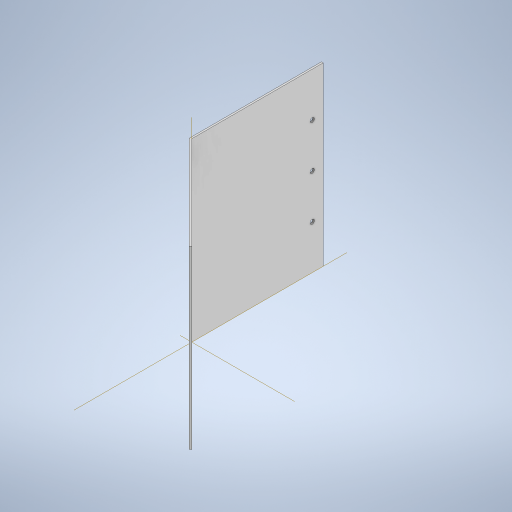
# Autodesk Inventor part: Thesis_part
Saved by Autodesk Inventor 2024 (Build 280153000, 153)
## iProperties
Created: 2024-02-06
Part Number: Thesis_part
Material: Generic
Document SubType Name: Modeling
Designer: Administrator
Density: 1 g/cm^3
Appearance: Default
Author: Administrator
Autodesk Inventor part; units mm, degrees
ref_plane "YZ Plane" through (0, 0, 0) normal (1, 0, 0) x (0, 1, 0)
ref_plane "XZ Plane" through (0, 0, 0) normal (0, 1, 0) x (-1, 0, 0)
ref_plane "XY Plane" through (0, 0, 0) normal (0, 0, 1) x (1, 0, 0)
sketch "Sketch2" plane through (0, 0, 0) normal (0, 1, 0) x (-1, 0, 0)
  line L0 (0, 0) -> (0, -149.1716)
  line L1 (-105.4802, 105.4802) -> (0, 0)
  line L2 (2, 0.8284) -> (2, -149.1716)
  line L3 (-104.066, 106.8944) -> (2, 0.8284)
  line L4 (-104.066, 106.8944) -> (-105.4802, 105.4802)
  line L5 (0, -149.1716) -> (2, -149.1716)
  line L6 (0, -200.3848) -> (0, 158.1076) projected
  dimension "d2" = 0
  dimension "d5" = 2
  dimension "d6" = 2
  dimension "d7" = 135
  dimension "d8" = 135
  dimension "d9" = 150
  dimension "d10" = 150
  dimension "d42" = 149.1716
  dimension "d43" = 149.1716
  constraints: 12 end point, 2 perpendicular, 1 parallel
  measures "d2" distance of point (0, 0) L0.start
  measures "d5" distance between parallel lines of L1 L3
  measures "d6" distance between parallel lines of L2 L0
  measures "d7" angle of L2 L3
  measures "d8" angle of L0 L1
  measures "d9" distance of L3.start L2.start
  measures "d10" distance of L2.start L2.end
  measures "d42" distance of L0.start L0.end
  measures "d43" distance of L1.start L0.start
extrude "Extrusion1" add sketch "Sketch2" along normal blind 200
sketch "Sketch3" plane through (0, 0, 0) normal (0.7071068, 0, -0.7071068) x (-0.7071068, 0, -0.7071068)
  circle A0 centre (-136.6716, 50) radius 2.5
  line L0 (-149.1716, 0) -> (-149.1716, 200) projected
  line L1 (-149.1716, 0) -> (0, 0) projected
  circle A1 centre (-136.6716, 100) radius 2.5
  circle A2 centre (-136.6716, 150) radius 2.5
  line L2 (-149.1716, 200) -> (0, 200) projected
  dimension "d11" = 12.5
  dimension "d13" = 5
  dimension "d14" = 5
  dimension "d16" = 5
  dimension "d17" = 12.5
  dimension "d19" = 12.5
  dimension "d20" = 50
  dimension "d21" = 50
  dimension "d24" = 50
  dimension "d25" = 50
  constraints: 3 centre point
  measures "d11" distance from line of L0 A0.centre
  measures "d13" diameter of A0
  measures "d14" diameter of A1
  measures "d16" diameter of A2
  measures "d17" distance from line of L0 A1.centre
  measures "d19" distance from line of L0 A2.centre
  measures "d20" distance from line of L1 A0.centre
  measures "d21" distance of A0.centre A1.centre
  measures "d24" distance from line of L2 A2.centre
  measures "d25" distance of A2.centre A1.centre
extrude "Extrusion2" cut sketch "Sketch3" against normal blind 3
sketch "Sketch4" plane through (0, 0, 0) normal (1, 0, 0) x (0, 0, -1)
  line L0 (149.1716, 0) -> (149.1716, 200) projected
  line L1 (0, 200) -> (149.1716, 200) projected
  line L2 (0, 0) -> (149.1716, 0) projected
  point P0 (136.6716, 150)
  point P1 (136.6716, 100)
  point P2 (136.6716, 50)
  dimension "d28" = 12.5
  dimension "d29" = 12.5
  dimension "d30" = 12.5
  dimension "d31" = 50
  dimension "d32" = 50
  dimension "d33" = 50
  dimension "d34" = 50
  measures "d28" distance from line of L0 point (136.672, 150)
  measures "d29" distance from line of L0 point (136.672, 100)
  measures "d30" distance from line of L0 point (136.672, 50)
  measures "d31" distance of point (136.672, 100) point (136.672, 50)
  measures "d32" distance of point (136.672, 150) point (136.672, 100)
  measures "d33" distance from line of L1 point (136.672, 150)
  measures "d34" distance from line of L2 point (136.672, 50)
hole "Hole1" at (0, 150, -136.6716) at (0, 100, -136.6716) at (0, 50, -136.6716) direction (-1, 0, 0) diameter 5 end through all
body "Solid1"
